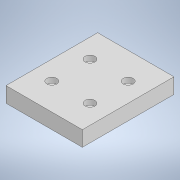
# Autodesk Inventor part: 26_Laser_carriage
Saved by Autodesk Inventor 2022.2 (Build 262287010, 287A)
## iProperties
Created: 2022-05-02
Part Number: 26_Laser_carriage
Material: Generisch
Document SubType Name: Modeling
Designer: MXBD
Density: 1 g/cm^3
Appearance: Vorgabe
Author: MXBD
Autodesk Inventor part; units mm, degrees
ref_plane "YZ Plane" through (0, 0, 0) normal (1, 0, 0) x (0, 1, 0)
ref_plane "XZ Plane" through (0, 0, 0) normal (0, 1, 0) x (-1, 0, 0)
ref_plane "XY Plane" through (0, 0, 0) normal (0, 0, 1) x (1, 0, 0)
sketch "Skizze1" plane through (0, 0, 0) normal (0, 1, 0) x (-1, 0, 0)
  line L0 (0, -42) -> (0, 42) projected
  line L1 (-35, 0) -> (35, 0) projected
  line L2 (-25, 30) -> (25, 30)
  line L3 (25, 30) -> (25, -30)
  line L4 (25, -30) -> (-25, -30)
  line L5 (-25, -30) -> (-25, 30)
  line L6 (-25, 30) -> (25, -30) construction
  line L7 (25, 30) -> (-25, -30) construction
  point P0 (0, 0)
  dimension "d0" = 50
  dimension "d1" = 60
  constraints: 12 end point, 2 midpoint, 2 parallel, 1 horizontal, 1 perpendicular
  measures "d0" distance of L3.end L4.end
  measures "d1" distance of L2.end L3.end
extrude "Extrusion1" add sketch "Skizze1" along normal mid plane 10
sketch "Skizze2" plane through (0, 5, 0) normal (0, 1, 0) x (1, 0, 0)
  line L0 (0, 42) -> (0, -42) projected
  line L1 (35, 0) -> (-35, 0) projected
  point P0 (0, 0)
  point P1 (-12.5, -12.5)
  point P2 (-12.5, 12.5)
  point P3 (12.5, 12.5)
  point P4 (12.5, -12.5)
  dimension "d4" = 25
  dimension "d5" = 25
  constraints: 3 symmetric about line
  measures "d4" distance of point (-12.5, 12.5) point (-12.5, -12.5)
  measures "d5" distance of point (12.5, 12.5) point (-12.5, 12.5)
hole "Bohrung1" at (-12.5, 5, 12.5) at (-12.5, 5, -12.5) at (12.5, 5, -12.5) at (12.5, 5, 12.5) direction (0, -1, 0) diameter 3.4 end through all counterbore diameter 6.5 counterbore depth 3.4 clearance for "Inbusschraube ISO 4762" size "M3" standard "ISO"
